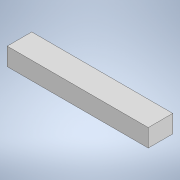
# Autodesk Inventor part: terminal_rail
Saved by Autodesk Inventor 2020 (Build 240168000, 168)
## iProperties
Created: 2019-12-04
Part Number: terminal_rail
Material: Generic
Document SubType Name: Modeling
Designer: Connor
Density: 1 g/cm^3
Appearance: Default
Author: Connor
Autodesk Inventor part; units mm, degrees
ref_plane "YZ Plane" through (0, 0, 0) normal (1, 0, 0) x (0, 1, 0)
ref_plane "XZ Plane" through (0, 0, 0) normal (0, 1, 0) x (-1, 0, 0)
ref_plane "XY Plane" through (0, 0, 0) normal (0, 0, 1) x (1, 0, 0)
sketch "Sketch1" plane through (0, 0, 0) normal (0, 1, 0) x (-1, 0, 0)
  line L0 (0, 0) -> (0, -22.098)
  line L1 (0, -22.098) -> (127, -22.098)
  line L2 (0, 0) -> (127, 0)
  line L3 (127, 0) -> (127, -22.098)
  dimension "d0" = 22.098
  dimension "d1" = 127
  constraints: 8 end point, 2 horizontal, 1 perpendicular, 1 vertical
  measures "d0" distance of L0.start L0.end
  measures "d1" distance of L0.end L1.end
extrude "Extrusion1" add sketch "Sketch1" along normal blind 16.002
body "Solid1"
